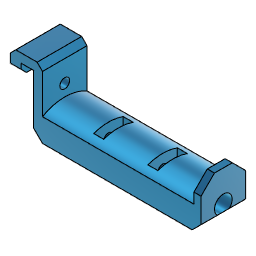
SpoolHolder B_1x_SN_BO (Autodesk Fusion 360 design; units mm, degrees)
Autodesk Fusion 360 part; units mm, degrees
note: some values were not read from the file. Set by a fixed rule: which sketch regions a step uses.
sketch "Sketch1" plane through (0, 0, 0) normal (0, 1, 0) x (1, 0, 0)
  line L0 (0, 0) -> (20, 0)
  line L1 (20, 0) -> (20, -20)
  line L2 (20, -20) -> (0, -20)
  line L3 (0, -20) -> (0, 0)
  line L4 (10, -20) -> (10, -25) construction
  line L5 (7, -25) -> (13, -25)
  line L6 (13, -25) -> (13, -14)
  line L7 (13, -14) -> (7, -14)
  line L8 (7, -14) -> (7, -25)
  line L9 (13, -25) -> (25, -25)
  line L10 (25, -25) -> (25, 0)
  line L11 (25, 0) -> (20, 0)
  dimension "d1" = 20
  dimension "d2" = 20
  dimension "d3" = 5
  dimension "d4" = 6
  dimension "d5" = 6
  dimension "d6" = 5
  constraint horizontal L0
  constraint vertical L1
  constraint horizontal L2
  constraint vertical L3
  constraint coincident L0.start L3.end
  constraint midpoint L2 L4.start
  constraint perpendicular L2 L4
  constraint horizontal L5
  constraint vertical L6
  constraint horizontal L7
  constraint vertical L8
  constraint midpoint L4.end L5
  constraint perpendicular L6 L9
  constraint perpendicular L9 L10
  constraint perpendicular L10 L11
  measures "d1" distance of L0.start L2.end
  measures "d2" distance of L0.start L0.end
  measures "d3" distance of L4.start L4.end
  measures "d4" distance of L2 L6.end
  measures "d5" distance of L5.start L5.end
  measures "d6" distance of L0.end L10.end
extrude "Extrude1" add sketch "Sketch1" along normal blind 25 contours L1 L2 L6 L9 L10 L11 | L2 L6 L7 L8 | L2 L5 L6 L8
hole "Hole3" at (20, 12.5, 10) direction (1, 0, 0) diameter 5.5 depth 11 tip angle 180
sketch "Sketch2" plane through (25, 0, 0) normal (1, 0, 0) x (0, 1, 0)
  line L0 (0, 25) -> (0, 0)
  line L1 (0, 0) -> (25, 0)
  line L2 (25, 0) -> (25, 25)
  line L3 (25, 25) -> (0, 25)
  arc A0 (25, 0) -> (0, 0) centre (12.5, -21.6506) ccw
  line L4 (0, 0) -> (0, -13)
  circle A1 centre (12.5, 10) radius 2.75
  line L5 (0, -13) -> (1.1286, -13)
  line L6 (1.1286, -13) -> (25, -13)
  line L7 (25, -13) -> (25, 0)
  dimension "d9" = 25
  dimension "d62" = 13
  constraint coincident L2 L1.end
  constraint coincident L0 L1.start
  constraint horizontal L0.end L1.end
  constraint coincident L0.end L1.start
  constraint perpendicular L1 L4
  constraint coincident L1.end L2.start
  constraint perpendicular L4 L5
  constraint perpendicular L2 L6
  constraint perpendicular L6 L7
  measures "d9" radius of A0
  measures "d62" distance of L1.end L6.end
extrude "Extrude2" add sketch "Sketch2" along normal blind 85 and the other way blind 5 contours L1 A0 | L1 L4 L5 L6 L7
sketch "Sketch3" plane through (110, 0, 0) normal (1, 0, 0) x (0, 1, 0)
  arc A0 (25, 0) -> (0, 0) centre (12.5, -21.6506) ccw
  line L0 (0, 0) -> (0, -13)
  line L1 (25, -13) -> (25, 0)
  line L2 (12.5, -16.6506) -> (12.5, 13.3494) construction
  line L3 (25, 13.3494) -> (25, 0)
  line L4 (25, 13.3494) -> (0, 13.3494)
  line L5 (0, 13.3494) -> (0, 0)
  line L6 (0, -13) -> (25, -13)
  dimension "d12" = 10
  dimension "d13" = 25
  constraint coincident A0.start L1.end
  constraint horizontal L4
  constraint midpoint L2.end L4
  constraint coincident A0.end L0.start
  measures "d12" distance of A0 L4
  measures "d13" distance of L3.start L4.end
extrude "Extrude3" add sketch "Sketch3" along normal blind 4
chamfer "Chamfer1" distance 3 angle 45 2 edges at (7, 12.5, 25) (25, 12.5, 25)
chamfer "Chamfer2" distance 3 angle 45 2 edges at (10, 0, 14) (10, 25, 14)
chamfer "Chamfer5" distance 7.5 angle 45 2 edges at (112, 0, 13.3494) (112, 25, 13.3494)
chamfer "Chamfer6" distance 5 angle 45 2 edges at (20, 12.5, -13) (114, 12.5, -13)
sketch "Sketch4" plane through (0, 0, 25) normal (0, 0, 1) x (-1, 0, 0)
  line L0 (-25, -25) -> (-25, 0)
  line L1 (-25, 0) -> (-110, 0)
  line L2 (-110, 0) -> (-110, -25)
  line L3 (-110, -25) -> (-25, -25)
  line L4 (-67.5, -25) -> (-67.5, 0) construction
  line L5 (-49.5, -25) -> (-85.5, -25)
  line L6 (-85.5, -25) -> (-85.5, 0)
  line L7 (-85.5, 0) -> (-49.5, 0)
  line L8 (-49.5, 0) -> (-49.5, -25)
  line L9 (-55.1, -25) -> (-79.9, -25)
  line L10 (-79.9, -25) -> (-79.9, 0)
  line L11 (-79.9, 0) -> (-55.1, 0)
  line L12 (-55.1, 0) -> (-55.1, -25)
  line L13 (-49.5, -12.5) -> (-85.5, -12.5) construction
  line L14 (-49.5, -20.75) -> (-85.5, -20.75)
  line L15 (-85.5, -20.75) -> (-85.5, -4.25)
  line L16 (-85.5, -4.25) -> (-49.5, -4.25)
  line L17 (-49.5, -4.25) -> (-49.5, -20.75)
  line L18 (-64.5, -20.75) -> (-70.5, -20.75)
  line L19 (-70.5, -20.75) -> (-70.5, -4.25)
  line L20 (-70.5, -4.25) -> (-64.5, -4.25)
  line L21 (-64.5, -4.25) -> (-64.5, -20.75)
  line L22 (-22, 0) -> (-22, -25)
  line L23 (-22, -25) -> (-10, -25)
  line L24 (-10, -25) -> (-10, 0)
  line L25 (-10, 0) -> (-22, 0)
  dimension "d22" = 36
  dimension "d23" = 5.6
  dimension "d24" = 20
  dimension "d25" = 16.5
  dimension "d29" = 21.5
  dimension "d31" = 6
  constraint midpoint L3 L4.start
  constraint midpoint L1 L4.end
  constraint horizontal L5
  constraint vertical L6
  constraint horizontal L7
  constraint vertical L8
  constraint coincident L1 L6.end
  constraint coincident L3 L5.start
  constraint midpoint L4.start L5
  constraint horizontal L9
  constraint vertical L10
  constraint horizontal L11
  constraint vertical L12
  constraint coincident L7 L10.end
  constraint coincident L5 L9.start
  constraint symmetric L4 L10.end L11.end
  constraint midpoint L8 L13.start
  constraint midpoint L6 L13.end
  constraint horizontal L14
  constraint vertical L15
  constraint horizontal L16
  constraint vertical L17
  constraint coincident L6 L15.end
  constraint coincident L8 L14.start
  constraint symmetric L13 L14.end L15.end
  constraint horizontal L18
  constraint vertical L19
  constraint horizontal L20
  constraint vertical L21
  constraint coincident L16 L19.end
  constraint coincident L14 L18.start
  constraint symmetric L4 L19.end L20.end
  measures "d22" distance of L5.start L5.end
  measures "d23" distance of L5.start L9.start
  measures "d25" distance of L14.end L15.end
  measures "d31" distance of L19.end L20.end
extrude "Extrude4" cut sketch "Sketch4" against normal blind 27 from surface at -5 contours L8 L12 L14 L16 L17 | L6 L10 L14 L15 L16
hole "Hole1" at (114, 12.5, -4.3253) direction (-1, 0, 0) diameter 5 depth 100 tip angle 118 counterbore diameter 10 counterbore depth 22
hole "Hole2" at (20, 12.5, -4.3253) direction (1, 0, 0) diameter 10 depth 23 tip angle 118
equation "d62 = 5 mm + 4 mm + 4 mm"
named bodies: "SpoolHolder B"
